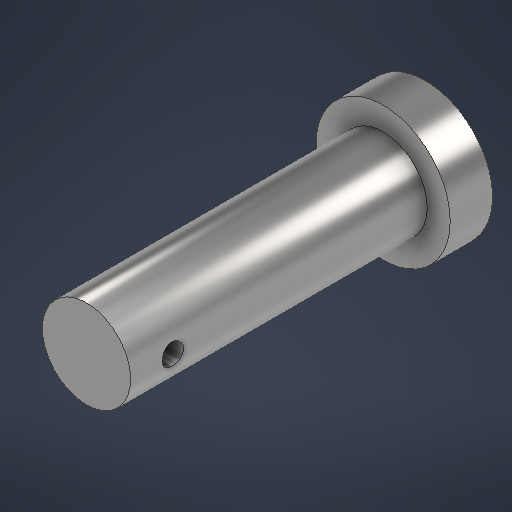
# Autodesk Inventor part: pin
Saved by Autodesk Inventor 2026.1 (Build 301233020, 233B)
## iProperties
Created: 2025-12-18
Part Number: pin
Material: Steel, Alloy
Document SubType Name: Modeling
Designer: kngob
Density: 7.73 g/cm^3
Appearance: Semi-Polished
Author: kngob
Autodesk Inventor part; units mm, degrees
ref_plane "YZ Plane" through (0, 0, 0) normal (1, 0, 0) x (0, 1, 0)
ref_plane "XZ Plane" through (0, 0, 0) normal (0, 1, 0) x (-1, 0, 0)
ref_plane "XY Plane" through (0, 0, 0) normal (0, 0, 1) x (1, 0, 0)
sketch "Sketch1" plane through (0, 0, 0) normal (0, 0, 1) x (1, 0, 0)
  circle A0 centre (0, 0) radius 19
  circle A1 centre (0, 0) radius 12.5
  dimension "d0" = 38
  dimension "d1" = 25
  constraints: 2 centre point, 2 coincident
  measures "d0" diameter of A0
  measures "d1" diameter of A1
extrude "Extrusion1" add sketch "Sketch1" along normal blind 96 contours A1
extrude "Extrusion2" add sketch "Sketch1" along normal blind 12
sketch "Sketch2" plane through (0, 0, 0) normal (1, 0, 0) x (0, 1, 0)
  circle A0 centre (0, 84) radius 3
  line L0 (12.5, 96) -> (-12.5, 96) projected
  point P0 (0, 0)
  dimension "d6" = 6
  dimension "d7" = 12
  constraints: 1 centre point
  measures "d6" diameter of A0
  measures "d7" distance from line of L0 A0.centre
extrude "Extrusion3" cut sketch "Sketch2" along normal through all both and the other way through all
body "Solid1"
